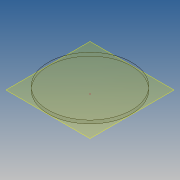
# Autodesk Inventor part: staklo
Saved by Autodesk Inventor 2014 (Build 180170000, 170)
## iProperties
Created: 2011-11-30
Part Number: staklo
Material: Generic
Document SubType Name: Modeling
Designer: slazh bliskovic
Density: 1 g/cm^3
Mass: 0.0613592 g
Surface Area: 2.65072 cm^2
Volume: 0.0613592 cm^3
Appearance: Clear - Light
Author: slazh bliskovic
Autodesk Inventor part; units mm, degrees
ref_plane "YZ Plane" through (0, 0, 0) normal (1, 0, 0) x (0, 1, 0)
ref_plane "XZ Plane" through (0, 0, 0) normal (0, 1, 0) x (-1, 0, 0)
ref_plane "XY Plane" through (0, 0, 0) normal (0, 0, 1) x (1, 0, 0)
sketch "Sketch1" plane through (0, 0, 0) normal (0, 0, 1) x (1, 0, 0)
  point P0 (0, 0)
ref_plane "Work Plane1" through (0, 0, 0.5) normal (0, 0, 1) x (1, 0, 0)
sketch "Sketch2" plane through (0, 0, 0.5) normal (0, 0, 1) x (1, 0, 0)
  circle A0 centre (0, 0) radius 6.25
  dimension "d0" = 12.5
  constraints: 1 centre point, 1 coincident
  measures "d0" diameter of A0
extrude "Extrusion1" add sketch "Sketch2" along normal blind 0.5
body "Solid1"
